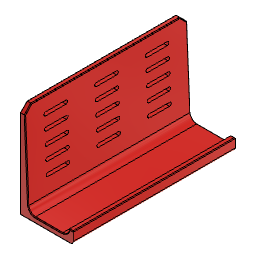
Phone Holder v4 (Autodesk Fusion 360 design; units mm, degrees)
Autodesk Fusion 360 part; units mm, degrees
sketch "Sketch1" plane through (0, 0, 0) normal (0, 1, 0) x (1, 0, 0)
  line L0 (0, 0) -> (49.4074, 0)
  line L1 (49.4074, 0) -> (49.4074, -10.795)
  line L2 (49.4074, -10.795) -> (45.5974, -10.795)
  line L3 (45.5974, -10.795) -> (45.5974, -4.445)
  line L4 (45.5974, -4.445) -> (7.4974, -4.445)
  line L5 (3.81, -88.9) -> (0, -88.9)
  line L6 (0, -88.9) -> (0, 0)
  line L7 (3.81, -88.9) -> (7.4974, -4.445)
  dimension "d3" = 4.445
  dimension "d10" = 6.35
  dimension "d12" = 92.5
  dimension "d13" = 3.81
  dimension "d15" = 88.9
  dimension "d16" = 38.1
  constraint coincident L0.start L6.end
  constraint horizontal L0
  constraint perpendicular L0 L1
  constraint perpendicular L1 L2
  constraint perpendicular L2 L3
  constraint perpendicular L3 L4
  constraint perpendicular L0 L6
  constraint equal L2 L5
  constraint horizontal L5
  measures "d3" distance of L0 L4
  measures "d10" distance of L2 L4
  measures "d12" angle of L4 L7
  measures "d13" distance of L5.start L5.end
  measures "d15" distance of L5.end L0.start
  measures "d16" distance of L3.end L4.end
extrude "Extrude1" add sketch "Sketch1" along normal blind 152.4
fillet "Fillet1" radius 6.35 2 edges at (45.5974, 76.2, 4.445) (7.4974, 76.2, 4.445)
sketch "Sketch2" plane through (0, 0, 0) normal (1, 0, 0) x (0, 1, 0)
  line L0 (0, 10.1925) -> (152.4, 10.1925)
  line L1 (152.4, 10.1925) -> (152.4, 88.6492)
  line L2 (152.4, 88.6492) -> (0, 88.6492)
  line L3 (0, 88.6492) -> (0, 10.1925)
  line L4 (19.05, 72.7742) -> (38.1, 72.7742)
  arc A0 (38.1, 72.7742) -> (38.1, 75.9492) centre (38.1, 74.3617) ccw
  line L5 (38.1, 75.9492) -> (19.05, 75.9492)
  arc A1 (19.05, 75.9492) -> (19.05, 72.7742) centre (19.05, 74.3617) ccw
  line L6 (19.05, 74.3617) -> (38.1, 74.3617) construction
  line L7 (0, 88.8154, -3.8064) -> (0, 88.6492, 0)
  line L8 (0, 88.6492) -> (152.4, 88.6492)
  line L9 (152.4, 88.6492, 0) -> (152.4, 88.8154, -3.8064)
  line L10 (152.4, 88.8154, -3.8064) -> (0, 88.8154, -3.8064)
  line L11 (19.05, 60.7092) -> (38.1, 60.7092)
  arc A2 (38.1, 60.7092) -> (38.1, 63.8842) centre (38.1, 62.2967) ccw
  line L12 (38.1, 63.8842) -> (19.05, 63.8842)
  arc A3 (19.05, 63.8842) -> (19.05, 60.7092) centre (19.05, 62.2967) ccw
  line L13 (19.05, 48.6442) -> (38.1, 48.6442)
  arc A4 (38.1, 48.6442) -> (38.1, 51.8192) centre (38.1, 50.2317) ccw
  line L14 (38.1, 51.8192) -> (19.05, 51.8192)
  arc A5 (19.05, 51.8192) -> (19.05, 48.6442) centre (19.05, 50.2317) ccw
  line L15 (19.05, 36.5792) -> (38.1, 36.5792)
  arc A6 (38.1, 36.5792) -> (38.1, 39.7542) centre (38.1, 38.1667) ccw
  line L16 (38.1, 39.7542) -> (19.05, 39.7542)
  arc A7 (19.05, 39.7542) -> (19.05, 36.5792) centre (19.05, 38.1667) ccw
  line L17 (19.05, 24.5142) -> (38.1, 24.5142)
  arc A8 (38.1, 24.5142) -> (38.1, 27.6892) centre (38.1, 26.1017) ccw
  line L18 (38.1, 27.6892) -> (19.05, 27.6892)
  arc A9 (19.05, 27.6892) -> (19.05, 24.5142) centre (19.05, 26.1017) ccw
  line L19 (0, 0) -> (0, 88.9)
  line L20 (0, 88.9) -> (152.4, 88.9)
  line L21 (152.4, 88.9) -> (152.4, 0)
  line L22 (152.4, 0) -> (0, 0)
  line L23 (76.2, 88.6492) -> (76.2, 35.56) construction
  arc A10 (133.35, 48.6442) -> (133.35, 51.8192) centre (133.35, 50.2317) ccw
  line L24 (133.35, 36.5792) -> (114.3, 36.5792)
  line L25 (114.3, 75.9492) -> (133.35, 75.9492)
  line L26 (114.3, 27.6892) -> (133.35, 27.6892)
  arc A11 (114.3, 27.6892) -> (114.3, 24.5142) centre (114.3, 26.1017) ccw
  line L27 (133.35, 74.3617) -> (114.3, 74.3617) construction
  line L28 (133.35, 60.7092) -> (114.3, 60.7092)
  line L29 (114.3, 63.8842) -> (133.35, 63.8842)
  line L30 (114.3, 51.8192) -> (133.35, 51.8192)
  arc A12 (133.35, 60.7092) -> (133.35, 63.8842) centre (133.35, 62.2967) ccw
  arc A13 (133.35, 24.5142) -> (133.35, 27.6892) centre (133.35, 26.1017) ccw
  line L31 (114.3, 39.7542) -> (133.35, 39.7542)
  line L32 (133.35, 24.5142) -> (114.3, 24.5142)
  arc A14 (114.3, 39.7542) -> (114.3, 36.5792) centre (114.3, 38.1667) ccw
  line L33 (133.35, 72.7742) -> (114.3, 72.7742)
  arc A15 (133.35, 72.7742) -> (133.35, 75.9492) centre (133.35, 74.3617) ccw
  arc A16 (114.3, 75.9492) -> (114.3, 72.7742) centre (114.3, 74.3617) ccw
  arc A17 (114.3, 63.8842) -> (114.3, 60.7092) centre (114.3, 62.2967) ccw
  line L34 (133.35, 48.6442) -> (114.3, 48.6442)
  arc A18 (133.35, 36.5792) -> (133.35, 39.7542) centre (133.35, 38.1667) ccw
  arc A19 (114.3, 51.8192) -> (114.3, 48.6442) centre (114.3, 50.2317) ccw
  line L35 (66.675, 75.9492) -> (85.725, 75.9492)
  line L36 (66.675, 51.8192) -> (85.725, 51.8192)
  arc A20 (66.675, 75.9492) -> (66.675, 72.7742) centre (66.675, 74.3617) ccw
  line L37 (66.675, 27.6892) -> (85.725, 27.6892)
  line L38 (85.725, 60.7092) -> (66.675, 60.7092)
  line L39 (85.725, 74.3617) -> (66.675, 74.3617) construction
  line L40 (85.725, 24.5142) -> (66.675, 24.5142)
  arc A21 (85.725, 72.7742) -> (85.725, 75.9492) centre (85.725, 74.3617) ccw
  arc A22 (66.675, 27.6892) -> (66.675, 24.5142) centre (66.675, 26.1017) ccw
  arc A23 (85.725, 48.6442) -> (85.725, 51.8192) centre (85.725, 50.2317) ccw
  line L41 (85.725, 48.6442) -> (66.675, 48.6442)
  arc A24 (66.675, 63.8842) -> (66.675, 60.7092) centre (66.675, 62.2967) ccw
  line L42 (66.675, 63.8842) -> (85.725, 63.8842)
  line L43 (85.725, 36.5792) -> (66.675, 36.5792)
  arc A25 (85.725, 24.5142) -> (85.725, 27.6892) centre (85.725, 26.1017) ccw
  arc A26 (85.725, 36.5792) -> (85.725, 39.7542) centre (85.725, 38.1667) ccw
  line L44 (85.725, 72.7742) -> (66.675, 72.7742)
  line L45 (66.675, 39.7542) -> (85.725, 39.7542)
  arc A27 (66.675, 51.8192) -> (66.675, 48.6442) centre (66.675, 50.2317) ccw
  arc A28 (85.725, 60.7092) -> (85.725, 63.8842) centre (85.725, 62.2967) ccw
  arc A29 (66.675, 39.7542) -> (66.675, 36.5792) centre (66.675, 38.1667) ccw
  point P0 (76.2, 75.9492)
  point P1 (76.2, 75.9492)
  dimension "d18" = 3.175
  dimension "d19" = 19.05
  dimension "d20" = 12.7
  dimension "d21" = 19.05
  dimension "d24" = 0
  dimension "d25" = -48.26
  constraint tangent L4 A0
  constraint tangent A0 L5
  constraint parallel L4 L5
  constraint tangent L5 A1
  constraint tangent L4 A1
  constraint parallel L2 L6
  constraint midpoint L8 L23.start
  constraint perpendicular L8 L23
  constraint symmetric L4.start L23 L33.start
  constraint symmetric L4.end L23 L33.end
  constraint symmetric A0.end L23 L25.start
  constraint symmetric L5.end L23 L25.end
  constraint symmetric A0 L23 A16
  constraint symmetric A1 L23 A15
  constraint symmetric L11.start L23 L28.start
  constraint symmetric L11.end L23 L28.end
  constraint symmetric A2.end L23 L29.start
  constraint symmetric A2 L23 A17
  constraint symmetric L12.end L23 L29.end
  constraint symmetric A3 L23 A12
  constraint symmetric L13.start L23 A10.start
  constraint symmetric L13.end L23 L34.end
  constraint symmetric A4.end L23 L30.start
  constraint symmetric A4 L23 A19
  constraint symmetric L14.end L23 A10.end
  constraint symmetric A5 L23 A10
  constraint symmetric L15.start L23 L24.start
  constraint symmetric L15.end L23 L24.end
  constraint symmetric A6.end L23 L31.start
  constraint symmetric A6 L23 A14
  constraint symmetric L16.end L23 L31.end
  constraint symmetric A7 L23 A18
  constraint symmetric L17.start L23 A13.start
  constraint symmetric L17.end L23 A11.end
  constraint symmetric A8.end L23 L26.start
  constraint symmetric A8 L23 A11
  constraint symmetric L18.end L23 L26.end
  constraint symmetric A9 L23 A13
  constraint midpoint L35 P1
  constraint coincident L23 P1
  measures "d18" distance of L4 L5
  measures "d19" distance of L3 A1.centre
  measures "d20" distance of L5 L8
  measures "d21" distance of A1.centre A0.centre
extrude "Extrude2" cut sketch "Sketch2" along normal blind 50.8 contours L4 A0 L5 A1 | L11 A2 L12 A3 | L13 A4 L14 A5 | L15 A6 L16 A7 | L17 A8 L18 A9 | A10 L30 L34 A19 | L24 L31 A14 A18 | L25 L33 A15 A16 | L26 A11 A13 L32 | L28 L29 A12 A17 | L35 A20 A21 L44 | L36 A23 L41 A27 | L37 L40 A22 A25 | L38 A24 L42 A28 | L43 A26 L45 A29
chamfer "Chamfer2" distance 6.35 angle 45 2 edges at (1.905, 0, 88.9) (1.905, 152.4, 88.9)
chamfer "Chamfer1" distance 0.635 angle 45 14 edges at (49.4074, 76.2, 10.795) (47.5024, 0, 10.795) (43.7375, 0, 6.3049) (26.4118, 0, 4.445) (9.1851, 0, 6.208) (5.6597, 0, 46.534) (3.81, 76.2, 88.9) (5.6597, 152.4, 46.534) (9.1851, 152.4, 6.208) (26.4118, 152.4, 4.445) (43.7375, 152.4, 6.3049) (47.5024, 152.4, 10.795) (3.9486, 3.175, 85.725) (3.9486, 149.225, 85.725)
fillet "Fillet2" radius 2.54 1 edges at (49.4074, 76.2, 0)
equation "d3 = thickness + 0.025 in"
equation "thickness = 0.15 in"
equation "d13 = thickness"
